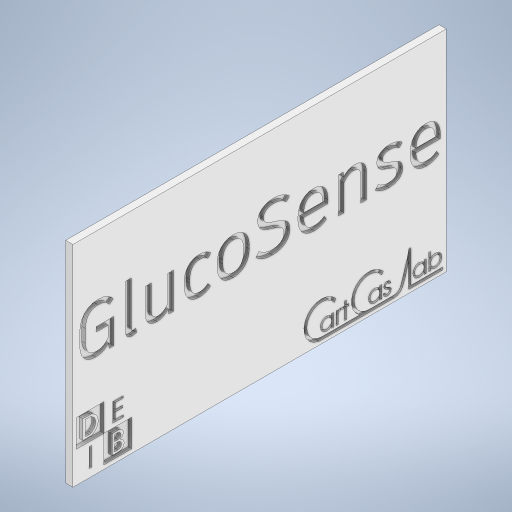
# Autodesk Inventor part: Targhetta
Saved by Autodesk Inventor 2023 (Build 270158000, 158)
## iProperties
Created: 2023-02-04
Part Number: Targhetta
Material: Generico
Document SubType Name: Modeling
Designer: Gabriele
Density: 1 g/cm^3
Appearance: Bianco
Author: Gabriele
Autodesk Inventor part; units mm, degrees
ref_plane "YZ Plane" through (0, 0, 0) normal (1, 0, 0) x (0, 1, 0)
ref_plane "XZ Plane" through (0, 0, 0) normal (0, 1, 0) x (-1, 0, 0)
ref_plane "XY Plane" through (0, 0, 0) normal (0, 0, 1) x (1, 0, 0)
sketch "Schizzo1" plane through (0, 0, 0) normal (1, 0, 0) x (0, 1, 0)
  line L0 (-29, 51.5) -> (29, 51.5)
  line L1 (29, 51.5) -> (29, -51.5)
  line L2 (29, -51.5) -> (-29, -51.5)
  line L3 (-29, -51.5) -> (-29, 51.5)
  line L4 (-29, 51.5) -> (29, -51.5) construction
  line L5 (29, 51.5) -> (-29, -51.5) construction
  point P0 (0, 0)
  dimension "d0" = 103
  dimension "d1" = 58
  constraints: 12 end point, 2 midpoint, 2 parallel, 1 horizontal, 1 perpendicular
  measures "d0" distance of L0.end L1.end
  measures "d1" distance of L0.start L0.end
extrude "Estrusione1" add sketch "Schizzo1" along normal blind 2
sketch "Schizzo2" plane through (2, 0, 0) normal (1, 0, 0) x (0, 0, -1)
  line L0 (-52.6017, 16.0027) -> (52.3954, 16.0027) construction
  line L1 (52.3954, 16.0027) -> (52.3954, -4.0809) construction
  line L2 (52.3954, -4.0809) -> (-52.6017, -4.0809) construction
  line L3 (-52.6017, -4.0809) -> (-52.6017, 16.0027) construction
  line L4 (-53.9264, -9.4627) -> (-32.0656, -9.4627) construction
  line L5 (-32.0656, -9.4627) -> (-32.0656, -31.3236) construction
  line L6 (-32.0656, -31.3236) -> (-53.9264, -31.3236) construction
  line L7 (-53.9264, -31.3236) -> (-53.9264, -9.4627) construction
  line L8 (-50.6221, -12.8348) -> (-35.2975, -12.8348)
  line L9 (-35.2975, -12.8348) -> (-35.2975, -27.8912)
  line L10 (-35.2975, -27.8912) -> (-50.6221, -27.8912)
  line L11 (-50.6221, -27.8912) -> (-50.6221, -12.8348)
  line L12 (-42.9598, -20.363) -> (-35.2975, -20.363)
  line L13 (-35.2975, -20.363) -> (-35.2975, -27.8912)
  line L14 (-35.2975, -27.8912) -> (-42.9598, -27.8912)
  line L15 (-42.9598, -27.8912) -> (-42.9598, -20.363)
  line L16 (-50.6221, -12.8348) -> (-42.9598, -12.8348)
  line L17 (-42.9598, -12.8348) -> (-42.9598, -20.363)
  line L18 (-42.9598, -20.363) -> (-50.6221, -20.363)
  line L19 (-50.6221, -20.363) -> (-50.6221, -12.8348)
  line L20 (-47.0581, -21.5952) -> (-46.3178, -21.5952)
  line L21 (-46.3178, -21.5952) -> (-46.3178, -26.7953)
  line L22 (-46.3178, -26.7953) -> (-47.0581, -26.7953)
  line L23 (-47.0581, -26.7953) -> (-47.0581, -21.5952)
  line L24 (-40.5401, -14.0622) -> (-39.8254, -14.0622)
  line L25 (-39.8254, -19.1638) -> (-40.5401, -19.1638)
  line L26 (-40.5401, -19.1638) -> (-40.5401, -14.0622)
  line L27 (-37.6814, -14.0622) -> (-39.8254, -14.0622)
  line L28 (-39.8254, -14.6096) -> (-37.6814, -14.6096)
  line L29 (-37.6814, -14.6096) -> (-37.6814, -14.0622)
  line L30 (-37.8335, -16.2443) -> (-39.8254, -16.2443)
  line L31 (-39.8254, -16.8525) -> (-37.8335, -16.8525)
  line L32 (-37.8335, -16.8525) -> (-37.8335, -16.2443)
  line L33 (-37.5902, -19.1638) -> (-39.8254, -19.1638)
  line L34 (-39.8254, -18.6316) -> (-37.5902, -18.6316)
  line L35 (-37.5902, -18.6316) -> (-37.5902, -19.1638)
  line L36 (-39.8254, -14.6096) -> (-39.8254, -16.2443)
  line L37 (-39.8254, -16.8525) -> (-39.8254, -18.6316)
  line L38 (-48.7669, -13.9939) -> (-48.7669, -19.1783)
  line L39 (-48.0762, -14.5149) -> (-48.0762, -18.6316)
  arc A0 (-46.4511, -18.5048) -> (-46.3958, -14.6584) centre (-47.3674, -16.5681) ccw
  line L40 (-48.0762, -14.5149) -> (-46.9944, -14.5149)
  line L41 (-48.0762, -18.6316) -> (-47.0156, -18.6316)
  arc A1 (-46.3958, -14.6584) -> (-46.9944, -14.5149) centre (-46.9944, -15.8349) ccw
  arc A2 (-47.0156, -18.6316) -> (-46.4511, -18.5048) centre (-47.0156, -17.3116) ccw
  line L42 (-40.7108, -21.5991) -> (-40.7108, -26.837)
  line L43 (-40.0437, -22.1315) -> (-40.0437, -23.8177)
  line L44 (-40.0437, -24.3455) -> (-40.0437, -26.2553)
  line L45 (-40.7108, -21.5991) -> (-38.8166, -21.5991)
  arc A3 (-38.46, -23.9953) -> (-38.8166, -21.5991) centre (-38.8121, -22.8231) ccw
  line L46 (-40.7108, -26.837) -> (-38.8102, -26.837)
  arc A4 (-38.8102, -26.837) -> (-38.46, -23.9953) centre (-38.8102, -25.3946) ccw
  line L47 (-40.0437, -22.1315) -> (-39.0607, -22.1315)
  line L48 (-40.0437, -23.8177) -> (-39.0607, -23.8177)
  arc A5 (-39.0607, -23.8177) -> (-39.0607, -22.1315) centre (-39.1165, -22.9746) ccw
  line L49 (-40.0437, -24.3455) -> (-39.0607, -24.3455)
  line L50 (-40.0437, -26.2553) -> (-39.0607, -26.2553)
  arc A6 (-39.0607, -26.2553) -> (-39.0607, -24.3455) centre (-39.0607, -25.3004) ccw
  line L51 (-48.7669, -13.9939) -> (-46.673, -13.9939)
  line L52 (-48.7669, -19.1783) -> (-46.6312, -19.1783)
  arc A7 (-46.0782, -19.0569) -> (-46.1598, -14.0977) centre (-47.2139, -16.5953) ccw
  arc A8 (-46.6312, -19.1783) -> (-46.0782, -19.0569) centre (-46.6312, -17.8583) ccw
  arc A9 (-46.1598, -14.0977) -> (-46.673, -13.9939) centre (-46.673, -15.3139) ccw
  line L53 (12.3073, -18.3154) -> (78.6844, -18.3154) construction
  line L54 (78.6844, -18.3154) -> (78.6844, -28.0734) construction
  line L55 (78.6844, -28.0734) -> (12.3073, -28.0734) construction
  line L56 (12.3073, -28.0734) -> (12.3073, -18.3154) construction
  arc A10 (20.6411, -20.9247) -> (17.2218, -27.3629) centre (17.1439, -23.1944) ccw
  arc A11 (21.0139, -20.1398) -> (16.4343, -28.0734) centre (17.1439, -23.1944) ccw
  arc A12 (33.6668, -20.8405) -> (30.472, -27.3629) centre (30.2193, -23.1955) ccw
  arc A13 (34.1255, -20.2465) -> (27.6526, -27.3629) centre (30.2193, -23.1955) ccw
  line L57 (21.0139, -20.1398) -> (20.6411, -20.9247)
  line L58 (34.1255, -20.2465) -> (33.6668, -20.8405)
  circle A14 centre (18.5203, -24.8878) radius 1.3335
  arc A15 (19.8538, -23.6888) -> (19.8538, -26.0868) centre (18.5203, -24.8878) ccw
  line L59 (16.4343, -28.0734) -> (36.9473, -28.0734)
  line L60 (17.066, -27.3629) -> (27.6526, -27.3629)
  line L61 (29.9665, -27.3629) -> (36.9473, -27.3629)
  line L62 (19.8538, -23.1955) -> (20.4033, -23.1955)
  line L63 (20.4033, -23.1955) -> (20.4033, -26.681)
  line L64 (20.4033, -26.681) -> (19.8538, -26.681)
  line L65 (19.8538, -26.681) -> (19.8538, -26.0868)
  line L66 (19.8538, -23.6888) -> (19.8538, -23.1955)
  line L67 (21.0978, -23.1955) -> (21.6469, -23.1955)
  line L68 (21.6469, -26.681) -> (21.0978, -26.681)
  line L69 (21.0978, -26.681) -> (21.0978, -23.1955)
  line L70 (22.4058, -23.1033) -> (22.4058, -23.5998)
  arc A16 (22.4058, -23.5998) -> (21.6469, -24.2703) centre (22.3226, -24.2703) ccw
  arc A17 (22.4058, -23.1033) -> (21.6469, -23.5096) centre (22.3588, -23.9272) ccw
  line L71 (21.6469, -23.1955) -> (21.6469, -23.5096)
  line L72 (21.6469, -24.2703) -> (21.6469, -26.681)
  line L73 (24.646, -23.1442) -> (24.646, -23.6558)
  line L74 (22.7069, -23.6558) -> (22.7069, -23.1442)
  line L75 (23.3731, -21.9894) -> (23.9397, -21.9894)
  line L76 (23.9397, -26.6273) -> (23.3731, -26.6273)
  line L77 (22.7069, -23.1442) -> (23.3731, -23.1442)
  line L78 (23.9397, -23.1442) -> (24.646, -23.1442)
  line L79 (23.3731, -26.6273) -> (23.3731, -23.6558)
  line L80 (23.3731, -23.1442) -> (23.3731, -21.9894)
  line L81 (24.646, -23.6558) -> (23.9397, -23.6558)
  line L82 (23.3731, -23.6558) -> (22.7069, -23.6558)
  line L83 (23.9397, -21.9894) -> (23.9397, -23.1442)
  line L84 (23.9397, -23.6558) -> (23.9397, -26.6273)
  line L85 (33.6719, -23.1483) -> (33.6719, -26.6339)
  line L86 (33.1224, -23.6416) -> (33.1224, -23.1483)
  line L87 (33.1224, -23.1483) -> (33.6719, -23.1483)
  line L88 (33.1224, -26.6339) -> (33.1224, -26.0396)
  line L89 (33.6719, -26.6339) -> (33.1224, -26.6339)
  circle A18 centre (31.789, -24.8406) radius 1.3335
  arc A19 (33.1224, -23.6416) -> (33.1224, -26.0396) centre (31.789, -24.8406) ccw
  line L90 (20.4033, -23.1955) -> (20.4033, -26.681)
  line L91 (19.8538, -23.6888) -> (19.8538, -23.1955)
  line L92 (19.8538, -23.1955) -> (20.4033, -23.1955)
  line L93 (19.8538, -26.681) -> (19.8538, -26.0868)
  line L94 (20.4033, -26.681) -> (19.8538, -26.681)
  circle A20 centre (18.5203, -24.8878) radius 1.3335
  arc A21 (19.8538, -23.6888) -> (19.8538, -26.0868) centre (18.5203, -24.8878) ccw
  line L95 (45.9489, -23.1483) -> (45.9489, -26.6339)
  line L96 (45.3994, -23.6416) -> (45.3994, -23.1483)
  line L97 (45.3994, -23.1483) -> (45.9489, -23.1483)
  line L98 (45.3994, -26.6339) -> (45.3994, -26.0396)
  line L99 (45.9489, -26.6339) -> (45.3994, -26.6339)
  circle A22 centre (44.0659, -24.8406) radius 1.3335
  arc A23 (45.3994, -23.6416) -> (45.3994, -26.0396) centre (44.0659, -24.8406) ccw
  line L100 (40.3597, -21.6337) -> (39.0206, -25.8248)
  arc A24 (36.9473, -27.3629) -> (39.0206, -25.8248) centre (37.1648, -25.4897) ccw
  arc A25 (40.3597, -21.6337) -> (41.1314, -18.4601) centre (8.0128, -12.0883) ccw
  arc A26 (36.9473, -28.0734) -> (39.4338, -26.5519) centre (37.1579, -25.625) ccw
  arc A27 (39.4338, -26.5519) -> (40.2757, -24.2985) centre (16.8627, -16.8354) ccw
  arc A28 (41.0648, -21.3179) -> (40.2757, -24.2985) centre (308.1135, -93.6127) ccw
  line L101 (41.0648, -21.3179) -> (41.0648, -27.8054)
  line L102 (41.3328, -28.0734) -> (50.2432, -28.0734)
  arc A29 (41.0648, -27.8054) -> (41.3328, -28.0734) centre (41.3328, -27.8054) ccw
  line L103 (41.7168, -18.4601) -> (41.7168, -27.0949)
  line L104 (41.9848, -27.3629) -> (50.2432, -27.3629)
  arc A30 (50.2432, -28.0734) -> (50.2432, -27.3629) centre (50.2432, -27.7182) ccw
  arc A31 (41.7168, -27.0949) -> (41.9848, -27.3629) centre (41.9848, -27.0949) ccw
  arc A32 (41.7168, -18.4601) -> (41.1314, -18.4601) centre (41.4241, -18.684) ccw
  circle A33 centre (48.474, -24.8406) radius 1.3182
  arc A34 (47.1558, -26.0551) -> (47.1558, -23.6261) centre (48.474, -24.8406) ccw
  line L105 (46.6816, -21.9894) -> (47.1558, -21.9894)
  line L106 (47.1558, -26.633) -> (46.6816, -26.633)
  line L107 (46.6816, -26.633) -> (46.6816, -21.9894)
  line L108 (47.1558, -21.9894) -> (47.1558, -23.6261)
  line L109 (47.1558, -26.0551) -> (47.1558, -26.633)
  arc A35 (36.1848, -23.9857) -> (34.2307, -24.028) centre (35.2086, -24.0478) ccw
  arc A36 (34.615, -25.5873) -> (35.7998, -25.4148) centre (35.2205, -25.591) ccw
  line L110 (34.615, -25.5873) -> (34.0596, -25.5873)
  arc A37 (34.0596, -25.5873) -> (36.2998, -25.6215) centre (35.1805, -25.5528) ccw
  arc A38 (36.2998, -25.6215) -> (35.8262, -24.8399) centre (35.4992, -25.5724) ccw
  arc A39 (35.6718, -23.9857) -> (34.7183, -24.2216) centre (35.1808, -24.0458) ccw
  line L111 (34.8519, -24.3675) -> (35.8262, -24.8399)
  line L112 (35.6718, -23.9857) -> (36.1848, -23.9857)
  arc A40 (34.2307, -24.028) -> (34.7765, -24.812) centre (35.1753, -23.9523) ccw
  line L113 (34.7765, -24.812) -> (35.5725, -25.19)
  arc A41 (35.7998, -25.4148) -> (35.5725, -25.19) centre (35.3648, -25.6274) ccw
  arc A42 (34.7183, -24.2216) -> (34.8519, -24.3675) centre (34.9688, -24.1263) ccw
  line L114 (-40.2267, -0.7994) -> (-41.5089, -0.7994)
  line L115 (-41.5089, -0.7994) -> (-41.6358, 0.5209)
  spline S0 degree 2 poles (-41.6358, 0.5209) (-42.2833, -0.19) (-44.086, -1.0279) (-45.2286, -1.0279) knots 0 0 0 1 2 2 2
  spline S1 degree 2 poles (-45.2286, -1.0279) (-46.5108, -1.0279) (-48.4913, 0.0766) (-49.6212, 2.1713) (-49.6212, 3.5805) knots 0 0 0 1 2 3 3 3
  line L116 (-49.6212, 3.5805) -> (-49.6212, 7.1479)
  spline S2 degree 2 poles (-49.6212, 7.1479) (-49.6212, 8.7348) (-48.4405, 11.1088) (-46.1681, 12.4291) (-44.5938, 12.4291) knots 0 0 0 1 2 3 3 3
  spline S3 degree 2 poles (-44.5938, 12.4291) (-43.0831, 12.4291) (-41.1026, 11.4262) (-40.3917, 10.4741) knots 0 0 0 1 2 2 2
  line L117 (-40.3917, 10.4741) -> (-41.4581, 9.6996)
  spline S4 degree 2 poles (-41.4581, 9.6996) (-42.0294, 10.436) (-43.464, 11.1469) (-44.5938, 11.1469) knots 0 0 0 1 2 2 2
  spline S5 degree 2 poles (-44.5938, 11.1469) (-46.2823, 11.1469) (-48.0343, 9.0395) (-48.0343, 7.186) knots 0 0 0 1 2 2 2
  line L118 (-48.0343, 7.186) -> (-48.0343, 3.6567)
  spline S6 degree 2 poles (-48.0343, 3.6567) (-48.0343, 2.0825) (-46.4093, 0.2543) (-44.9112, 0.2543) knots 0 0 0 1 2 2 2
  spline S7 degree 2 poles (-44.9112, 0.2543) (-43.8448, 0.2543) (-42.2579, 1.1684) (-41.7628, 2.0063) knots 0 0 0 1 2 2 2
  line L119 (-41.7628, 2.0063) -> (-41.7501, 4.9008)
  line L120 (-41.7501, 4.9008) -> (-45.0509, 4.9008)
  line L121 (-45.0509, 4.9008) -> (-45.0509, 6.183)
  line L122 (-45.0509, 6.183) -> (-40.2267, 6.183)
  line L123 (-40.2267, 6.183) -> (-40.2267, -0.7994)
  spline S8 degree 2 poles (-35.4278, 1.1176) (-35.4278, 0.6479) (-35.0851, 0.2416) (-34.6915, 0.2416) knots 0 0 0 1 2 2 2
  spline S9 degree 2 poles (-34.6915, 0.2416) (-34.5392, 0.2416) (-34.171, 0.3178) knots 0 0 0 1 1 1
  line L124 (-34.171, 0.3178) -> (-33.9679, -0.7994)
  spline S10 degree 2 poles (-33.9679, -0.7994) (-34.5392, -1.0279) (-35.0977, -1.0279) knots 0 0 0 1 1 1
  spline S11 degree 2 poles (-35.0977, -1.0279) (-35.9737, -1.0279) (-36.9893, -0.0504) (-36.9893, 0.851) knots 0 0 0 1 2 2 2
  line L125 (-36.9893, 0.851) -> (-36.9893, 12.9496)
  line L126 (-36.9893, 12.9496) -> (-35.4278, 12.9496)
  line L127 (-35.4278, 12.9496) -> (-35.4278, 1.1176)
  line L128 (-23.7608, 9.0014) -> (-23.7608, -0.7994)
  line L129 (-23.7608, -0.7994) -> (-25.0811, -0.7994)
  line L130 (-25.0811, -0.7994) -> (-25.2081, 0.4955)
  spline S12 degree 2 poles (-25.2081, 0.4955) (-25.8175, -0.2281) (-27.3917, -1.0279) (-28.3438, -1.0279) knots 0 0 0 1 2 2 2
  spline S13 degree 2 poles (-28.3438, -1.0279) (-29.6768, -1.0279) (-31.4415, 0.5971) (-31.4415, 1.9301) knots 0 0 0 1 2 2 2
  line L131 (-31.4415, 1.9301) -> (-31.4415, 9.0014)
  line L132 (-31.4415, 9.0014) -> (-29.88, 9.0014)
  line L133 (-29.88, 9.0014) -> (-29.88, 1.9809)
  spline S14 degree 2 poles (-29.88, 1.9809) (-29.88, 1.1557) (-28.9151, 0.2163) (-28.0518, 0.2163) knots 0 0 0 1 2 2 2
  spline S15 degree 2 poles (-28.0518, 0.2163) (-27.252, 0.2163) (-25.8175, 1.0795) (-25.3224, 1.8413) knots 0 0 0 1 2 2 2
  line L134 (-25.3224, 1.8413) -> (-25.3224, 9.0014)
  line L135 (-25.3224, 9.0014) -> (-23.7608, 9.0014)
  spline S16 degree 2 poles (-16.6007, -1.0279) (-17.921, -1.0279) (-19.838, 0.1909) (-20.8409, 2.3237) (-20.8409, 3.6948) knots 0 0 0 1 2 3 3 3
  line L136 (-20.8409, 3.6948) -> (-20.8409, 4.5073)
  spline S17 degree 2 poles (-20.8409, 4.5073) (-20.8409, 6.6274) (-18.6065, 9.2299) (-16.588, 9.2299) knots 0 0 0 1 2 2 2
  spline S18 degree 2 poles (-16.588, 9.2299) (-15.6358, 9.2299) (-14.1251, 8.6205) (-13.4649, 7.9858) knots 0 0 0 1 2 2 2
  line L137 (-13.4649, 7.9858) -> (-14.2647, 7.1098)
  spline S19 degree 2 poles (-14.2647, 7.1098) (-14.7472, 7.5541) (-15.8263, 7.9858) (-16.5245, 7.9858) knots 0 0 0 1 2 2 2
  spline S20 degree 2 poles (-16.5245, 7.9858) (-17.8448, 7.9858) (-19.2794, 6.183) (-19.2794, 4.5454) knots 0 0 0 1 2 2 2
  line L138 (-19.2794, 4.5454) -> (-19.2794, 3.6821)
  spline S21 degree 2 poles (-19.2794, 3.6821) (-19.2794, 2.0444) (-17.8829, 0.2163) (-16.5626, 0.2163) knots 0 0 0 1 2 2 2
  spline S22 degree 2 poles (-16.5626, 0.2163) (-15.8897, 0.2163) (-14.8233, 0.6733) (-14.2647, 1.0541) knots 0 0 0 1 2 2 2
  line L139 (-14.2647, 1.0541) -> (-13.5538, 0.0766)
  spline S23 degree 2 poles (-13.5538, 0.0766) (-14.1632, -0.4312) (-15.7628, -1.0279) (-16.6007, -1.0279) knots 0 0 0 1 2 2 2
  spline S24 degree 2 poles (-7.295, 9.2299) (-5.8858, 9.2299) (-3.9054, 8.0366) (-2.8643, 5.9672) (-2.8643, 4.6215) knots 0 0 0 1 2 3 3 3
  line L140 (-2.8643, 4.6215) -> (-2.8643, 3.644)
  spline S25 degree 2 poles (-2.8643, 3.644) (-2.8643, 2.2856) (-3.9054, 0.1655) (-5.8858, -1.0279) (-7.295, -1.0279) knots 0 0 0 1 2 3 3 3
  spline S26 degree 2 poles (-7.295, -1.0279) (-9.4151, -1.0279) (-11.7257, 1.562) (-11.7257, 3.644) knots 0 0 0 1 2 2 2
  line L141 (-11.7257, 3.644) -> (-11.7257, 4.6215)
  spline S27 degree 2 poles (-11.7257, 4.6215) (-11.7257, 5.9672) (-10.6974, 8.0366) (-8.7169, 9.2299) (-7.295, 9.2299) knots 0 0 0 1 2 3 3 3
  spline S28 degree 2 poles (-7.295, 7.9858) (-8.6788, 7.9858) (-10.1642, 6.2211) (-10.1642, 4.6469) knots 0 0 0 1 2 2 2
  line L142 (-10.1642, 4.6469) -> (-10.1642, 3.6567)
  spline S29 degree 2 poles (-10.1642, 3.6567) (-10.1642, 2.019) (-8.6788, 0.2163) (-7.295, 0.2163) knots 0 0 0 1 2 2 2
  spline S30 degree 2 poles (-7.295, 0.2163) (-5.9239, 0.2163) (-4.4259, 2.0444) (-4.4259, 3.6567) knots 0 0 0 1 2 2 2
  line L143 (-4.4259, 3.6567) -> (-4.4259, 4.6469)
  spline S31 degree 2 poles (-4.4259, 4.6469) (-4.4259, 6.2211) (-5.9239, 7.9858) (-7.295, 7.9858) knots 0 0 0 1 2 2 2
  spline S32 degree 2 poles (3.5468, -1.0279) (1.9726, -1.0279) (-0.2364, -0.1519) (-1.0362, 0.6352) knots 0 0 0 1 2 2 2
  line L144 (-1.0362, 0.6352) -> (-0.1856, 1.6381)
  spline S33 degree 2 poles (-0.1856, 1.6381) (0.4491, 1.1684) (1.3632, 0.6479) (2.62, 0.3178) (3.5341, 0.3178) knots 0 0 0 1 2 3 3 3
  spline S34 degree 2 poles (3.5341, 0.3178) (4.5878, 0.3178) (6.0224, 0.9653) (6.6952, 1.9682) (6.6952, 2.5014) knots 0 0 0 1 2 3 3 3
  line L145 (6.6952, 2.5014) -> (6.6952, 2.8061)
  spline S35 degree 2 poles (6.6952, 2.8061) (6.6952, 3.6567) (5.6669, 4.6215) (4.372, 5.0532) knots 0 0 0 1 2 2 2
  line L146 (4.372, 5.0532) -> (2.4931, 5.6625)
  spline S36 degree 2 poles (2.4931, 5.6625) (0.8935, 6.183) (-0.5411, 7.7573) (-0.5411, 8.8364) knots 0 0 0 1 2 2 2
  line L147 (-0.5411, 8.8364) -> (-0.5411, 9.2426)
  spline S37 degree 2 poles (-0.5411, 9.2426) (-0.5411, 10.0678) (0.4872, 11.5151) (2.4931, 12.4291) (3.8896, 12.4291) knots 0 0 0 1 2 3 3 3
  spline S38 degree 2 poles (3.8896, 12.4291) (6.4921, 12.4291) (8.2314, 10.7407) knots 0 0 0 1 1 1
  line L148 (8.2314, 10.7407) -> (7.3808, 9.8266)
  spline S39 degree 2 poles (7.3808, 9.8266) (6.5429, 10.5248) (4.9687, 11.1469) (3.9023, 11.1469) knots 0 0 0 1 2 2 2
  spline S40 degree 2 poles (3.9023, 11.1469) (2.9374, 11.1469) (1.6552, 10.5883) (1.0585, 9.7123) (1.0585, 9.2426) knots 0 0 0 1 2 3 3 3
  line L149 (1.0585, 9.2426) -> (1.0585, 8.8745)
  spline S41 degree 2 poles (1.0585, 8.8745) (1.0585, 8.2397) (2.1757, 7.3002) (3.4071, 6.9067) knots 0 0 0 1 2 2 2
  line L150 (3.4071, 6.9067) -> (5.0956, 6.3481)
  spline S42 degree 2 poles (5.0956, 6.3481) (6.6317, 5.8657) (8.2821, 4.3295) (8.2821, 2.9584) knots 0 0 0 1 2 2 2
  line L151 (8.2821, 2.9584) -> (8.2821, 2.4887)
  spline S43 degree 2 poles (8.2821, 2.4887) (8.2821, 1.4985) (7.1396, -0.0884) (4.9814, -1.0279) (3.5468, -1.0279) knots 0 0 0 1 2 3 3 3
  spline S44 degree 2 poles (18.8573, 4.5454) (18.8573, 3.9741) (18.8065, 3.6059) knots 0 0 0 1 1 1
  line L152 (18.8065, 3.6059) -> (12.1161, 3.6059)
  spline S45 degree 2 poles (12.1161, 3.6059) (12.1161, 1.9555) (13.6903, 0.2163) (15.163, 0.2163) knots 0 0 0 1 2 2 2
  spline S46 degree 2 poles (15.163, 0.2163) (15.9374, 0.2163) (17.1689, 0.6733) (17.829, 1.0922) knots 0 0 0 1 2 2 2
  line L153 (17.829, 1.0922) -> (18.4257, 0.1147)
  spline S47 degree 2 poles (18.4257, 0.1147) (17.8036, -0.3931) (16.0517, -1.0279) (15.0868, -1.0279) knots 0 0 0 1 2 2 2
  spline S48 degree 2 poles (15.0868, -1.0279) (13.6903, -1.0279) (11.6464, 0.1909) (10.5673, 2.2983) (10.5673, 3.644) knots 0 0 0 1 2 3 3 3
  line L154 (10.5673, 3.644) -> (10.5673, 4.6088)
  spline S49 degree 2 poles (10.5673, 4.6088) (10.5673, 5.9038) (11.5956, 8.0239) (13.5253, 9.2299) (14.8075, 9.2299) knots 0 0 0 1 2 3 3 3
  spline S50 degree 2 poles (14.8075, 9.2299) (16.6991, 9.2299) (18.8573, 6.7543) (18.8573, 4.5454) knots 0 0 0 1 2 2 2
  spline S51 degree 2 poles (17.4482, 4.85) (17.4482, 6.31) (16.0644, 7.9858) (14.8075, 7.9858) knots 0 0 0 1 2 2 2
  spline S52 degree 2 poles (14.8075, 7.9858) (13.538, 7.9858) (12.1542, 6.2719) (12.1161, 4.7358) knots 0 0 0 1 2 2 2
  line L155 (12.1161, 4.7358) -> (17.4482, 4.7358)
  line L156 (17.4482, 4.7358) -> (17.4482, 4.85)
  spline S53 degree 2 poles (26.2714, 9.2299) (27.6806, 9.2299) (29.4452, 7.5161) (29.4452, 5.9799) knots 0 0 0 1 2 2 2
  line L157 (29.4452, 5.9799) -> (29.4452, -0.7994)
  line L158 (29.4452, -0.7994) -> (27.8837, -0.7994)
  line L159 (27.8837, -0.7994) -> (27.8837, 5.8276)
  spline S54 degree 2 poles (27.8837, 5.8276) (27.8837, 6.9321) (26.8681, 7.9858) (25.9286, 7.9858) knots 0 0 0 1 2 2 2
  spline S55 degree 2 poles (25.9286, 7.9858) (24.3163, 7.9858) (23.2753, 6.3735) knots 0 0 0 1 1 1
  line L160 (23.2753, 6.3735) -> (23.2753, -0.7994)
  line L161 (23.2753, -0.7994) -> (21.7138, -0.7994)
  line L162 (21.7138, -0.7994) -> (21.7138, 9.0014)
  line L163 (21.7138, 9.0014) -> (23.0341, 9.0014)
  line L164 (23.0341, 9.0014) -> (23.161, 7.7827)
  spline S56 degree 2 poles (23.161, 7.7827) (24.2782, 9.2299) (26.2714, 9.2299) knots 0 0 0 1 1 1
  spline S57 degree 2 poles (35.7167, -1.0279) (34.5614, -1.0279) (32.6317, -0.355) (31.8827, 0.2543) knots 0 0 0 1 2 2 2
  line L165 (31.8827, 0.2543) -> (32.6698, 1.2446)
  spline S58 degree 2 poles (32.6698, 1.2446) (33.9267, 0.2163) (35.5898, 0.2163) knots 0 0 0 1 1 1
  spline S59 degree 2 poles (35.5898, 0.2163) (36.6562, 0.2163) (37.8495, 0.9526) (37.8495, 1.6508) knots 0 0 0 1 2 2 2
  line L166 (37.8495, 1.6508) -> (37.8495, 1.8032)
  spline S60 degree 2 poles (37.8495, 1.8032) (37.8495, 2.4379) (37.0751, 3.1235) (36.0087, 3.4916) knots 0 0 0 1 2 2 2
  line L167 (36.0087, 3.4916) -> (34.7138, 3.936)
  spline S61 degree 2 poles (34.7138, 3.936) (33.4823, 4.3676) (32.3398, 5.5102) (32.3398, 6.3862) knots 0 0 0 1 2 2 2
  line L168 (32.3398, 6.3862) -> (32.3398, 6.7416)
  spline S62 degree 2 poles (32.3398, 6.7416) (32.3398, 7.4653) (33.2284, 8.5952) (34.8026, 9.2299) (35.7929, 9.2299) knots 0 0 0 1 2 3 3 3
  spline S63 degree 2 poles (35.7929, 9.2299) (36.8085, 9.2299) (38.6112, 8.6205) (39.3222, 8.0366) knots 0 0 0 1 2 2 2
  line L169 (39.3222, 8.0366) -> (38.5605, 7.1098)
  spline S64 degree 2 poles (38.5605, 7.1098) (37.8368, 7.5922) (36.5673, 7.9858) (35.8056, 7.9858) knots 0 0 0 1 2 2 2
  spline S65 degree 2 poles (35.8056, 7.9858) (34.8915, 7.9858) (33.8886, 7.3129) (33.8886, 6.7543) knots 0 0 0 1 2 2 2
  line L170 (33.8886, 6.7543) -> (33.8886, 6.5893)
  spline S66 degree 2 poles (33.8886, 6.5893) (33.8886, 6.0688) (34.6757, 5.4086) (35.6913, 5.0532) knots 0 0 0 1 2 2 2
  line L171 (35.6913, 5.0532) -> (36.9989, 4.5834)
  spline S67 degree 2 poles (36.9989, 4.5834) (38.205, 4.1645) (39.411, 3.0219) (39.411, 1.9809) knots 0 0 0 1 2 2 2
  line L172 (39.411, 1.9809) -> (39.411, 1.6381)
  spline S68 degree 2 poles (39.411, 1.6381) (39.411, 0.394) (37.3163, -1.0279) (35.7167, -1.0279) knots 0 0 0 1 2 2 2
  spline S69 degree 2 poles (49.8466, 4.5454) (49.8466, 3.9741) (49.7958, 3.6059) knots 0 0 0 1 1 1
  line L173 (49.7958, 3.6059) -> (43.1054, 3.6059)
  spline S70 degree 2 poles (43.1054, 3.6059) (43.1054, 1.9555) (44.6796, 0.2163) (46.1523, 0.2163) knots 0 0 0 1 2 2 2
  spline S71 degree 2 poles (46.1523, 0.2163) (46.9267, 0.2163) (48.1581, 0.6733) (48.8183, 1.0922) knots 0 0 0 1 2 2 2
  line L174 (48.8183, 1.0922) -> (49.4149, 0.1147)
  spline S72 degree 2 poles (49.4149, 0.1147) (48.7929, -0.3931) (47.0409, -1.0279) (46.0761, -1.0279) knots 0 0 0 1 2 2 2
  spline S73 degree 2 poles (46.0761, -1.0279) (44.6796, -1.0279) (42.6356, 0.1909) (41.5565, 2.2983) (41.5565, 3.644) knots 0 0 0 1 2 3 3 3
  line L175 (41.5565, 3.644) -> (41.5565, 4.6088)
  spline S74 degree 2 poles (41.5565, 4.6088) (41.5565, 5.9038) (42.5849, 8.0239) (44.5146, 9.2299) (45.7968, 9.2299) knots 0 0 0 1 2 3 3 3
  spline S75 degree 2 poles (45.7968, 9.2299) (47.6884, 9.2299) (49.8466, 6.7543) (49.8466, 4.5454) knots 0 0 0 1 2 2 2
  spline S76 degree 2 poles (48.4374, 4.85) (48.4374, 6.31) (47.0536, 7.9858) (45.7968, 7.9858) knots 0 0 0 1 2 2 2
  spline S77 degree 2 poles (45.7968, 7.9858) (44.5273, 7.9858) (43.1435, 6.2719) (43.1054, 4.7358) knots 0 0 0 1 2 2 2
  line L176 (43.1054, 4.7358) -> (48.4374, 4.7358)
  line L177 (48.4374, 4.7358) -> (48.4374, 4.85)
  point P0 (0, 0)
  point P1 (-46.7909, -18.6316)
  point P2 (-46.7548, -14.5149)
  point P3 (-46.4513, -13.9939)
  point P4 (-46.3909, -19.1783)
  point P5 (30.4125, -23.1472)
  point P6 (30.4125, -23.1472)
  point P7 (17.1439, -23.1944)
  point P8 (17.1439, -23.1944)
  point P9 (42.6894, -23.1472)
  point P10 (42.6894, -23.1472)
  point P11 (41.0648, -28.0734)
  point P12 (34.7765, -24.3309)
  point P13 (19.8538, -23.6888)
  dimension "d4" = 1.32
  dimension "d5" = 1.32
  dimension "d6" = 0.268
  dimension "d7" = 0.268
  dimension "d8" = 0.268
  constraints: 204 end point, 83 point on circle, 43 centre point, 42 parallel, 31 horizontal, 24 tangent, 19 perpendicular, 14 point on line, 10 coincident, 7 vertical, 2 equal radius, 4 other
  measures "d4" radius of A1
  measures "d5" radius of A8
  measures "d6" radius of A29
  measures "d7" radius of A31
  measures "d8" radius of A42
extrude "Estrusione2" cut sketch "Schizzo2" against normal blind 1 contours L8 L17 L18 L11 | L12 L9 L10 L15 | L20 L21 L22 L23 | L24 L27 L29 L28 L36 L30 L32 L31 L37 L34 L35 L33 L25 L26 | L40 A1 A0 A2 L41 L39 | L47 A5 L48 L43 | L49 A6 L50 L44 | A10 L60 A13 L58 A12 L61 A24 L100 A25 A32 L103 A31 L104 A30 L102 A29 L101 A28 A27 A26 L59 A11 L57 | L66 L62 L63 L64 L65 A15 | L67 L71 A17 L70 A16 L72 L68 L69 | L73 L81 L84 L76 L79 L82 L74 L77 L80 L75 L83 L78 | L85 L89 L88 A19 L86 L87 | L95 L99 L98 A23 L96 L97 | L109 L106 L107 L105 L108 A34 | L112 A39 A42 L111 A38 A37 L110 A36 A41 L113 A40 A35 | L114 L115 S0 S1 L116 S2 S3 L117 S4 S5 L118 S6 S7 L119 L120 L121 L122 L123 | S8 S9 L124 S10 S11 L125 L126 L127 | L128 L129 L130 S12 S13 L131 L132 L133 S14 S15 L134 L135 | S16 L136 S17 S18 L137 S19 S20 L138 S21 S22 L139 S23 | S24 L140 S25 S26 L141 S27 | S32 L144 S33 S34 L145 S35 L146 S36 L147 S37 S38 L148 S39 S40 L149 S41 L150 S42 L151 S43 | S44 L152 S45 S46 L153 S47 S48 L154 S49 S50 | S53 L157 L158 L159 S54 S55 L160 L161 L162 L163 L164 S56 | S57 L165 S58 S59 L166 S60 L167 S61 L168 S62 S63 L169 S64 S65 L170 S66 L171 S67 L172 S68 | S69 L173 S70 S71 L174 S72 S73 L175 S74 S75
